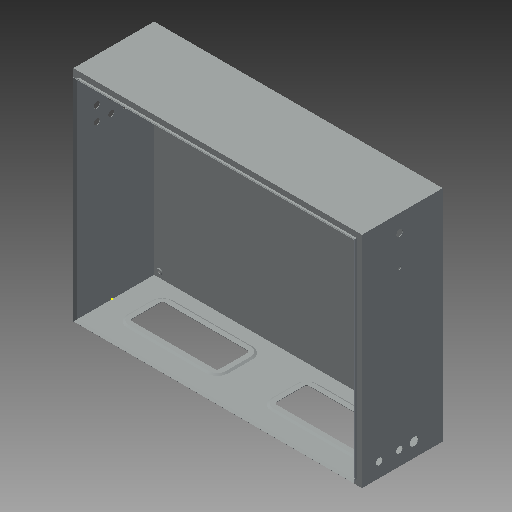
# Autodesk Inventor part: 1130_01_00 (2)
Saved by Autodesk Inventor 2019.3 (Build 233278000, 278)
## iProperties
Category: PARTsolutions
Company: RITTAL
Created: 2018-11-14
Part Number: 1130_01_00 (2)
Material: Generic
Catalog Web Link: www.cadenas.de
Description: Gehäusekorpus AE-Gehäusekorpus AE
Vendor: RITTAL
Document SubType Name: Modeling
Designer: psadmin
Manufacturer: RITTAL
Mass: 2682.24 g
Surface Area: 35840.6 cm^2
Volume: 2682.24 cm^3
Density: 1 g/cm^3
Appearance: PSOLRGB-195-201-196
PSOL_IDENT_0: {$CADENAS_DATA\23d-libs\rittal_usa\schaltschranksys\kompakt_schaltschr\ae\parts_ae\gehaeusekorpus_ae
PSOL_IDENT_1: .prj},204 {VTYP=3D},{NB=1130_01_00 (2)},{LINA=1130_01_00 (2)},{NN=Gehäusekorpus AE},{DATE=08.11.2018
PSOL_IDENT_2: 06:46:30},{GEOMDATE=18.08.2014 07:27:00},{VERSION=v140818072938},{LINEID=220},{WBVAR=DETAIL},{WBNUM
PSOL_IDENT_3: ERIC=DETAIL}  {NB=1130_01_00 (2)},{LINA=1130_01_00 (2)},{KT=DUMMY},{BEST=1130},{VER1=1},{VER2=1},{BE
PSOL_IDENT_4: Z1=MIN},{BEZ2=MIN},{BEZ3=MIN},{VER=1},{SS=1.50},{DETAIL=2},{A=1000.000},{B=760.000},{C=300.000},{D=3
PSOL_IDENT_5: 03.000},{E=113.000},{F=70.000},{G=30.000},{H=705.000},{I=667.200},{K=730.000},{P=905.000},{Q=944.000
PSOL_IDENT_6: },{R=495.000},{S=755.000},{T=616.400},{U=675.000},{V=27.000},{W=698.000},{X=0.000},{Y=0.000},{B1=100
PSOL_IDENT_7: 0},{H1=760},{T1=300},{F1=944},{G1=730},{S1=3.0},{GEW=56.0},{VERS=2},{GG=10.000},{AA=17.000},{BB=7.00
PSOL_IDENT_8: 0},{CC=10.000},{RR=31.000}
NN: Gehäusekorpus AE
NT: Gehäusekorpus AE
NB: 1130_01_00 (2)
NBSYN: $BEST._01_00 ($DETAIL.)
LINA: 1130_01_00 (2)
BEST: 1130
VER1: 1
VER2: 1
BEZ1: 0
BEZ2: 0
BEZ3: 0
VER: 1
SS: 1.5
DETAIL: 2
A: 1000
B: 760
C: 300
D: 303
E: 113
F: 70
G: 30
H: 705
I: 667.2
K: 730
P: 905
Q: 944
R: 495
S: 755
T: 616.4
U: 675
V: 27
W: 698
X: 0
Y: 0
B1: 1000
H1: 760
T1: 300
F1: 944
G1: 730
S1: 3
GEW: 56
VERS: 2
GG: 10
AA: 17
BB: 7
CC: 10
RR: 31
SUPPLIER: RITTAL
ARTICLENO: 1130_01_00 (2)
BOMINFO: 1130_01_00 (2)
CREATOR: CADENAS GmbH
Title: 1130_01_00 (2)
Author: Cadenas PARTsolutions
Comments: Gehäusekorpus AE
Autodesk Inventor part; units mm, degrees
sketch "Sketch_10" plane through (0, 0, 0) normal (0, 1, 0) x (-1, 0, 0)
  line L0 (500, 130) -> (-500, 130)
  line L1 (-500, 130) -> (-500, -150)
  line L2 (-500, -150) -> (500, -150)
  line L3 (500, -150) -> (500, 130)
  constraints: 8 end point
extrude "Extrusion1" add sketch "Sketch_10" along normal blind 760
sketch "Skizze_4" plane through (0, 0, 0) normal (1, 0, 0) x (0, 0, -1)
  line L0 (-300, 741) -> (-300, 19)
  line L1 (-300, 19) -> (0, 19)
  line L2 (0, 19) -> (0, 741)
  line L3 (0, 741) -> (-300, 741)
  constraints: 8 end point
extrude "Extrusion2" cut sketch "Skizze_4" along normal mid plane 961
sketch "Sketch_9" plane through (0, 0, 0) normal (1, 0, 0) x (0, 1, 0)
  line L0 (758.5, 128.5) -> (1.5, 128.5)
  line L1 (1.5, 128.5) -> (1.5, -148.5)
  line L2 (1.5, -148.5) -> (758.5, -148.5)
  line L3 (758.5, -148.5) -> (758.5, 128.5)
  constraints: 8 end point
extrude "Extrusion3" cut sketch "Sketch_9" along normal mid plane 997
sketch "Skizze_6" plane through (0, 0, 0) normal (1, 0, 0) x (0, 0, -1)
  line L0 (-144.3113, 14.6427) -> (-143.4081, 13.4441)
  line L1 (-143.4081, 13.4441) -> (-136.225, 18.5)
  line L2 (-136.225, 18.5) -> (-128.5, 18.5)
  line L3 (-128.5, 18.5) -> (-128.5, 20)
  line L4 (-128.5, 20) -> (-136.7, 20)
  line L5 (-136.7, 20) -> (-144.3113, 14.6427)
  constraints: 12 end point
extrude "Extrusion4" add sketch "Skizze_6" along normal mid plane 974.4
sketch "Skizze_7" plane through (0, 0, 0) normal (1, 0, 0) x (0, 0, -1)
  line L0 (-144.3113, 745.3573) -> (-136.7, 740)
  line L1 (-136.7, 740) -> (-128.5, 740)
  line L2 (-128.5, 740) -> (-128.5, 741.5)
  line L3 (-128.5, 741.5) -> (-136.225, 741.5)
  line L4 (-136.225, 741.5) -> (-143.4081, 746.5559)
  line L5 (-143.4081, 746.5559) -> (-144.3113, 745.3573)
  constraints: 12 end point
extrude "Extrusion5" add sketch "Skizze_7" along normal mid plane 973
sketch "Skizze_8" plane through (0, 380, 0) normal (0, 1, 0) x (1, 0, 0)
  line L0 (480, -136.7) -> (485.3573, -144.3113)
  line L1 (485.3573, -144.3113) -> (487.5552, -144.3113)
  line L2 (487.5552, -144.3113) -> (487.5552, -128.5)
  line L3 (487.5552, -128.5) -> (480, -128.5)
  line L4 (480, -128.5) -> (480, -136.7)
  constraints: 10 end point
extrude "Extrusion6" add sketch "Skizze_8" along normal mid plane 737.4
sketch "Skizze_9" plane through (0, 380, 0) normal (0, 1, 0) x (1, 0, 0)
  line L0 (-487.5552, -144.3113) -> (-485.3573, -144.3113)
  line L1 (-485.3573, -144.3113) -> (-480, -136.7)
  line L2 (-480, -136.7) -> (-480, -128.5)
  line L3 (-480, -128.5) -> (-487.5552, -128.5)
  line L4 (-487.5552, -128.5) -> (-487.5552, -144.3113)
  constraints: 10 end point
extrude "Extrusion7" add sketch "Skizze_9" along normal mid plane 737.4
sketch "Skizze_20" plane through (0, 0, 0) normal (1, 0, 0) x (0, 0, -1)
  line L0 (-439.6277, 761.5) -> (-439.6277, -1.5)
  line L1 (-439.6277, -1.5) -> (-130, -1.5)
  line L2 (-130, -1.5) -> (-130, 18.5)
  line L3 (-130, 18.5) -> (-136.225, 18.5)
  line L4 (-136.225, 18.5) -> (-143.4081, 13.4441)
  line L5 (-143.4081, 13.4441) -> (-419.6277, 380)
  line L6 (-419.6277, 380) -> (-143.4081, 746.5559)
  line L7 (-143.4081, 746.5559) -> (-136.225, 741.5)
  line L8 (-136.225, 741.5) -> (-130, 741.5)
  line L9 (-130, 741.5) -> (-130, 761.5)
  line L10 (-130, 761.5) -> (-439.6277, 761.5)
  constraints: 22 end point
extrude "Extrusion8" cut sketch "Skizze_20" along normal mid plane 1973
sketch "Skizze_21" plane through (0, 380, 0) normal (0, 1, 0) x (1, 0, 0)
  line L0 (-501.5, -530.0542) -> (501.5, -530.0542)
  line L1 (501.5, -530.0542) -> (501.5, -130)
  line L2 (501.5, -130) -> (481.5, -130)
  line L3 (481.5, -130) -> (481.5, -136.225)
  line L4 (481.5, -136.225) -> (486.5559, -143.4081)
  line L5 (486.5559, -143.4081) -> (0, -510.0542)
  line L6 (0, -510.0542) -> (-486.5559, -143.4081)
  line L7 (-486.5559, -143.4081) -> (-481.5, -136.225)
  line L8 (-481.5, -136.225) -> (-481.5, -130)
  line L9 (-481.5, -130) -> (-501.5, -130)
  line L10 (-501.5, -130) -> (-501.5, -530.0542)
  constraints: 22 end point
extrude "Extrusion9" cut sketch "Skizze_21" along normal mid plane 752.4
sketch "Skizze_28" plane through (0, 0, 0) normal (0, 1, 0) x (1, 0, 0)
  arc A0 (-432.9449, -16.4449) -> (-384.9449, -64.4449) centre (-384.9449, -16.4449) ccw
  line L0 (-384.9449, -64.4449) -> (-115.0551, -64.4449)
  arc A1 (-115.0551, -64.4449) -> (-67.0551, -16.4449) centre (-115.0551, -16.4449) ccw
  line L1 (-67.0551, -16.4449) -> (-67.0551, 63.4449)
  arc A2 (-67.0551, 63.4449) -> (-115.0551, 111.4449) centre (-115.0551, 63.4449) ccw
  line L2 (-115.0551, 111.4449) -> (-384.9449, 111.4449)
  arc A3 (-384.9449, 111.4449) -> (-432.9449, 63.4449) centre (-384.9449, 63.4449) ccw
  line L3 (-432.9449, 63.4449) -> (-432.9449, -16.4449)
  constraints: 8 end point, 8 point on circle, 4 centre point
extrude "Extrusion10" cut sketch "Skizze_28" along normal blind 1.5
sketch "Skizze_29" plane through (0, 0, -23.5) normal (0, 0, 1) x (1, 0, 0)
  line L0 (-102.5, 5.5) -> (-102.5, 4)
  line L1 (-102.5, 4) -> (-81.9019, 4)
  line L2 (-81.9019, 4) -> (-74.9737, 0)
  line L3 (-74.9737, 0) -> (-66.7551, 0)
  line L4 (-66.7551, 0) -> (-66.7551, 1.5)
  line L5 (-66.7551, 1.5) -> (-74.5718, 1.5)
  line L6 (-74.5718, 1.5) -> (-81.5, 5.5)
  line L7 (-81.5, 5.5) -> (-102.5, 5.5)
  constraints: 16 end point
extrude "Extrusion11" add sketch "Skizze_29" along normal mid plane 85
sketch "Skizze_30" plane through (0, 0, -23.5) normal (0, 0, 1) x (1, 0, 0)
  line L0 (-433.2449, 1.5) -> (-433.2449, 0)
  line L1 (-433.2449, 0) -> (-425.3263, 0)
  line L2 (-425.3263, 0) -> (-418.3981, 4)
  line L3 (-418.3981, 4) -> (-397.8, 4)
  line L4 (-397.8, 4) -> (-397.8, 5.5)
  line L5 (-397.8, 5.5) -> (-418.8, 5.5)
  line L6 (-418.8, 5.5) -> (-425.7282, 1.5)
  line L7 (-425.7282, 1.5) -> (-433.2449, 1.5)
  constraints: 16 end point
extrude "Extrusion12" add sketch "Skizze_30" along normal mid plane 85
sketch "Skizze_31" plane through (0, 0, -66) normal (0, 0, 1) x (1, 0, 0)
  line L0 (-112.5, -50) -> (-112.5, 50)
  line L1 (-102.5, 5.5) -> (-102.5, 4)
  line L2 (-102.5, 4) -> (-81.9019, 4)
  line L3 (-81.9019, 4) -> (-74.9737, 0)
  line L4 (-74.9737, 0) -> (-66.7551, 0)
  line L5 (-66.7551, 0) -> (-66.7551, 1.5)
  line L6 (-66.7551, 1.5) -> (-74.5718, 1.5)
  line L7 (-74.5718, 1.5) -> (-81.5, 5.5)
  line L8 (-81.5, 5.5) -> (-102.5, 5.5)
  constraints: 18 end point
revolve "Revolution1" add sketch "Skizze_31" angle 90 about axis through (-112.5, -50, -66) along (0, 1, 0)
sketch "Skizze_32" plane through (0, 0, -66) normal (0, 0, 1) x (1, 0, 0)
  line L0 (-387.5, 4) -> (-387.5, -4)
  line L1 (-433.2449, 1.5) -> (-433.2449, 0)
  line L2 (-433.2449, 0) -> (-425.0263, 0)
  line L3 (-425.0263, 0) -> (-418.0981, 4)
  line L4 (-418.0981, 4) -> (-397.5, 4)
  line L5 (-397.5, 4) -> (-397.5, 5.5)
  line L6 (-397.5, 5.5) -> (-418.5, 5.5)
  line L7 (-418.5, 5.5) -> (-425.4282, 1.5)
  line L8 (-425.4282, 1.5) -> (-433.2449, 1.5)
  constraints: 18 end point
revolve "Revolution2" add sketch "Skizze_32" angle 90 about axis through (-387.5, 4, -66) along (0, -1, 0)
sketch "Skizze_33" plane through (0, 0, 19) normal (0, 0, 1) x (1, 0, 0)
  line L0 (-112.5, -50) -> (-112.5, 50)
  line L1 (-102.5, 5.5) -> (-102.5, 4)
  line L2 (-102.5, 4) -> (-81.9019, 4)
  line L3 (-81.9019, 4) -> (-74.9737, 0)
  line L4 (-74.9737, 0) -> (-66.7551, 0)
  line L5 (-66.7551, 0) -> (-66.7551, 1.5)
  line L6 (-66.7551, 1.5) -> (-74.5718, 1.5)
  line L7 (-74.5718, 1.5) -> (-81.5, 5.5)
  line L8 (-81.5, 5.5) -> (-102.5, 5.5)
  constraints: 18 end point
revolve "Revolution3" add sketch "Skizze_33" angle 90 about axis through (-112.5, -50, 19) along (0, -1, 0)
sketch "Skizze_34" plane through (0, 0, 19) normal (0, 0, 1) x (1, 0, 0)
  line L0 (-387.5, 4) -> (-387.5, -4)
  line L1 (-433.2449, 1.5) -> (-433.2449, 0)
  line L2 (-433.2449, 0) -> (-425.0263, 0)
  line L3 (-425.0263, 0) -> (-418.0981, 4)
  line L4 (-418.0981, 4) -> (-397.5, 4)
  line L5 (-397.5, 4) -> (-397.5, 5.5)
  line L6 (-397.5, 5.5) -> (-418.5, 5.5)
  line L7 (-418.5, 5.5) -> (-425.4282, 1.5)
  line L8 (-425.4282, 1.5) -> (-433.2449, 1.5)
  constraints: 18 end point
revolve "Revolution4" add sketch "Skizze_34" angle 90 about axis through (-387.5, 4, 19) along (0, 1, 0)
sketch "Skizze_35" plane through (-250, 0, 0) normal (1, 0, 0) x (0, 0, -1)
  line L0 (76, 5.5) -> (76, 4)
  line L1 (76, 4) -> (96.5981, 4)
  line L2 (96.5981, 4) -> (103.5263, 0)
  line L3 (103.5263, 0) -> (111.7449, 0)
  line L4 (111.7449, 0) -> (111.7449, 1.5)
  line L5 (111.7449, 1.5) -> (103.9282, 1.5)
  line L6 (103.9282, 1.5) -> (97, 5.5)
  line L7 (97, 5.5) -> (76, 5.5)
  constraints: 16 end point
extrude "Extrusion13" add sketch "Skizze_35" along normal mid plane 275
sketch "Skizze_36" plane through (-250, 0, 0) normal (1, 0, 0) x (0, 0, -1)
  line L0 (-64.7449, 1.5) -> (-64.7449, 0)
  line L1 (-64.7449, 0) -> (-56.5263, 0)
  line L2 (-56.5263, 0) -> (-49.5981, 4)
  line L3 (-49.5981, 4) -> (-29, 4)
  line L4 (-29, 4) -> (-29, 5.5)
  line L5 (-29, 5.5) -> (-50, 5.5)
  line L6 (-50, 5.5) -> (-56.9282, 1.5)
  line L7 (-56.9282, 1.5) -> (-64.7449, 1.5)
  constraints: 16 end point
extrude "Extrusion14" add sketch "Skizze_36" along normal mid plane 275
sketch "Skizze_105" plane through (0, 5.5, 0) normal (0, 1, 0) x (1, 0, 0)
  line L0 (-401.5, -33) -> (-98.5, -33)
  line L1 (-98.5, -33) -> (-98.5, 80)
  line L2 (-98.5, 80) -> (-401.5, 80)
  line L3 (-401.5, 80) -> (-401.5, -33)
  constraints: 8 end point
extrude "Extrusion15" add sketch "Skizze_105" against normal blind 1.5
sketch "Skizze_106" plane through (0, 5.5, 0) normal (0, 1, 0) x (1, 0, 0)
  arc A0 (-401.5, -25) -> (-393.5, -33) centre (-393.5, -25) ccw
  line L0 (-393.5, -33) -> (-106.5, -33)
  arc A1 (-106.5, -33) -> (-98.5, -25) centre (-106.5, -25) ccw
  line L1 (-98.5, -25) -> (-98.5, 72)
  arc A2 (-98.5, 72) -> (-106.5, 80) centre (-106.5, 72) ccw
  line L2 (-106.5, 80) -> (-393.5, 80)
  arc A3 (-393.5, 80) -> (-401.5, 72) centre (-393.5, 72) ccw
  line L3 (-401.5, 72) -> (-401.5, -25)
  constraints: 8 end point, 8 point on circle, 4 centre point
extrude "Extrusion16" cut sketch "Skizze_106" against normal blind 1.5
sketch "Skizze_37" plane through (0, 0, 0) normal (0, 1, 0) x (1, 0, 0)
  arc A0 (67.0551, -16.4449) -> (115.0551, -64.4449) centre (115.0551, -16.4449) ccw
  line L0 (115.0551, -64.4449) -> (384.9449, -64.4449)
  arc A1 (384.9449, -64.4449) -> (432.9449, -16.4449) centre (384.9449, -16.4449) ccw
  line L1 (432.9449, -16.4449) -> (432.9449, 63.4449)
  arc A2 (432.9449, 63.4449) -> (384.9449, 111.4449) centre (384.9449, 63.4449) ccw
  line L2 (384.9449, 111.4449) -> (115.0551, 111.4449)
  arc A3 (115.0551, 111.4449) -> (67.0551, 63.4449) centre (115.0551, 63.4449) ccw
  line L3 (67.0551, 63.4449) -> (67.0551, -16.4449)
  constraints: 8 end point, 8 point on circle, 4 centre point
extrude "Extrusion17" cut sketch "Skizze_37" along normal blind 1.5
sketch "Skizze_38" plane through (0, 0, -23.5) normal (0, 0, 1) x (1, 0, 0)
  line L0 (397.5, 5.5) -> (397.5, 4)
  line L1 (397.5, 4) -> (418.0981, 4)
  line L2 (418.0981, 4) -> (425.0263, 0)
  line L3 (425.0263, 0) -> (433.2449, 0)
  line L4 (433.2449, 0) -> (433.2449, 1.5)
  line L5 (433.2449, 1.5) -> (425.4282, 1.5)
  line L6 (425.4282, 1.5) -> (418.5, 5.5)
  line L7 (418.5, 5.5) -> (397.5, 5.5)
  constraints: 16 end point
extrude "Extrusion18" add sketch "Skizze_38" along normal mid plane 85
sketch "Skizze_39" plane through (0, 0, -23.5) normal (0, 0, 1) x (1, 0, 0)
  line L0 (66.7551, 1.5) -> (66.7551, 0)
  line L1 (66.7551, 0) -> (74.9737, 0)
  line L2 (74.9737, 0) -> (81.9019, 4)
  line L3 (81.9019, 4) -> (102.5, 4)
  line L4 (102.5, 4) -> (102.5, 5.5)
  line L5 (102.5, 5.5) -> (81.5, 5.5)
  line L6 (81.5, 5.5) -> (74.5718, 1.5)
  line L7 (74.5718, 1.5) -> (66.7551, 1.5)
  constraints: 16 end point
extrude "Extrusion19" add sketch "Skizze_39" along normal mid plane 85
sketch "Skizze_40" plane through (0, 0, -66) normal (0, 0, 1) x (1, 0, 0)
  line L0 (387.5, -4) -> (387.5, 4)
  line L1 (397.5, 5.5) -> (397.5, 4)
  line L2 (397.5, 4) -> (418.0981, 4)
  line L3 (418.0981, 4) -> (425.0263, 0)
  line L4 (425.0263, 0) -> (433.2449, 0)
  line L5 (433.2449, 0) -> (433.2449, 1.5)
  line L6 (433.2449, 1.5) -> (425.4282, 1.5)
  line L7 (425.4282, 1.5) -> (418.5, 5.5)
  line L8 (418.5, 5.5) -> (397.5, 5.5)
  constraints: 18 end point
revolve "Revolution5" add sketch "Skizze_40" angle 90 about axis through (387.5, -4, -66) along (0, 1, 0)
sketch "Skizze_41" plane through (0, 0, -66) normal (0, 0, 1) x (1, 0, 0)
  line L0 (112.5, 4) -> (112.5, -4)
  line L1 (66.7551, 1.5) -> (66.7551, 0)
  line L2 (66.7551, 0) -> (74.9737, 0)
  line L3 (74.9737, 0) -> (81.9019, 4)
  line L4 (81.9019, 4) -> (102.5, 4)
  line L5 (102.5, 4) -> (102.5, 5.5)
  line L6 (102.5, 5.5) -> (81.5, 5.5)
  line L7 (81.5, 5.5) -> (74.5718, 1.5)
  line L8 (74.5718, 1.5) -> (66.7551, 1.5)
  constraints: 18 end point
revolve "Revolution6" add sketch "Skizze_41" angle 90 about axis through (112.5, 4, -66) along (0, -1, 0)
sketch "Skizze_42" plane through (0, 0, 19) normal (0, 0, 1) x (1, 0, 0)
  line L0 (387.5, -4) -> (387.5, 4)
  line L1 (397.5, 5.5) -> (397.5, 4)
  line L2 (397.5, 4) -> (418.0981, 4)
  line L3 (418.0981, 4) -> (425.0263, 0)
  line L4 (425.0263, 0) -> (433.2449, 0)
  line L5 (433.2449, 0) -> (433.2449, 1.5)
  line L6 (433.2449, 1.5) -> (425.4282, 1.5)
  line L7 (425.4282, 1.5) -> (418.5, 5.5)
  line L8 (418.5, 5.5) -> (397.5, 5.5)
  constraints: 18 end point
revolve "Revolution7" add sketch "Skizze_42" angle 90 about axis through (387.5, -4, 19) along (0, -1, 0)
sketch "Skizze_43" plane through (0, 0, 19) normal (0, 0, 1) x (1, 0, 0)
  line L0 (112.5, 4) -> (112.5, -4)
  line L1 (66.7551, 1.5) -> (66.7551, 0)
  line L2 (66.7551, 0) -> (74.9737, 0)
  line L3 (74.9737, 0) -> (81.9019, 4)
  line L4 (81.9019, 4) -> (102.5, 4)
  line L5 (102.5, 4) -> (102.5, 5.5)
  line L6 (102.5, 5.5) -> (81.5, 5.5)
  line L7 (81.5, 5.5) -> (74.5718, 1.5)
  line L8 (74.5718, 1.5) -> (66.7551, 1.5)
  constraints: 18 end point
revolve "Revolution8" add sketch "Skizze_43" angle 90 about axis through (112.5, 4, 19) along (0, 1, 0)
sketch "Skizze_44" plane through (250, 0, 0) normal (1, 0, 0) x (0, 0, -1)
  line L0 (76, 5.5) -> (76, 4)
  line L1 (76, 4) -> (96.5981, 4)
  line L2 (96.5981, 4) -> (103.5263, 0)
  line L3 (103.5263, 0) -> (111.7449, 0)
  line L4 (111.7449, 0) -> (111.7449, 1.5)
  line L5 (111.7449, 1.5) -> (103.9282, 1.5)
  line L6 (103.9282, 1.5) -> (97, 5.5)
  line L7 (97, 5.5) -> (76, 5.5)
  constraints: 16 end point
extrude "Extrusion20" add sketch "Skizze_44" along normal mid plane 275
sketch "Skizze_45" plane through (250, 0, 0) normal (1, 0, 0) x (0, 0, -1)
  line L0 (-64.7449, 1.5) -> (-64.7449, 0)
  line L1 (-64.7449, 0) -> (-56.5263, 0)
  line L2 (-56.5263, 0) -> (-49.5981, 4)
  line L3 (-49.5981, 4) -> (-29, 4)
  line L4 (-29, 4) -> (-29, 5.5)
  line L5 (-29, 5.5) -> (-50, 5.5)
  line L6 (-50, 5.5) -> (-56.9282, 1.5)
  line L7 (-56.9282, 1.5) -> (-64.7449, 1.5)
  constraints: 16 end point
extrude "Extrusion21" add sketch "Skizze_45" along normal mid plane 275
sketch "Skizze_107" plane through (0, 5.5, 0) normal (0, 1, 0) x (1, 0, 0)
  line L0 (98.5, -33) -> (401.5, -33)
  line L1 (401.5, -33) -> (401.5, 80)
  line L2 (401.5, 80) -> (98.5, 80)
  line L3 (98.5, 80) -> (98.5, -33)
  constraints: 8 end point
extrude "Extrusion22" add sketch "Skizze_107" against normal blind 1.5
sketch "Skizze_108" plane through (0, 5.5, 0) normal (0, 1, 0) x (1, 0, 0)
  arc A0 (98.5, -25) -> (106.5, -33) centre (106.5, -25) ccw
  line L0 (106.5, -33) -> (393.5, -33)
  arc A1 (393.5, -33) -> (401.5, -25) centre (393.5, -25) ccw
  line L1 (401.5, -25) -> (401.5, 72)
  arc A2 (401.5, 72) -> (393.5, 80) centre (393.5, 72) ccw
  line L2 (393.5, 80) -> (106.5, 80)
  arc A3 (106.5, 80) -> (98.5, 72) centre (106.5, 72) ccw
  line L3 (98.5, 72) -> (98.5, -25)
  constraints: 8 end point, 8 point on circle, 4 centre point
extrude "Extrusion23" cut sketch "Skizze_108" against normal blind 1.5
sketch "Sketch32" plane through (500, 0, -150) normal (0, 0, -1) x (-1, 0, 0)
  point P0 (20, 20)
hole "Hole1" at (480, 20, -150) direction (0, 0, 1) diameter 24 depth 1.5
sketch "Sketch33" plane through (500, 0, -150) normal (0, 0, -1) x (-1, 0, 0)
  point P0 (20, 740)
hole "Hole2" at (480, 740, -150) direction (0, 0, 1) diameter 24 depth 1.5
sketch "Skizze_68" plane through (480, 0, 0) normal (1, 0, 0) x (0, 0, -1)
  line L0 (150, 20) -> (148.5, 20)
  line L1 (146.5, 28.6213) -> (146.5, 24.35)
  line L2 (146.5, 24.35) -> (148, 24.35)
  line L3 (148, 24.35) -> (148, 28)
  line L4 (148, 28) -> (150, 30)
  line L5 (150, 30) -> (150, 32.5)
  line L6 (150, 32.5) -> (148.5, 32.5)
  line L7 (148.5, 32.5) -> (148.5, 30.6213)
  line L8 (148.5, 30.6213) -> (146.5, 28.6213)
  constraints: 18 end point
revolve "Revolution9" add sketch "Skizze_68" angle 360 about axis through (480, 20, -150) along (0, 0, -1)
sketch "Skizze_71" plane through (480, 0, 0) normal (1, 0, 0) x (0, 0, -1)
  line L0 (150, 740) -> (148.5, 740)
  line L1 (146.5, 748.6213) -> (146.5, 744.35)
  line L2 (146.5, 744.35) -> (148, 744.35)
  line L3 (148, 744.35) -> (148, 748)
  line L4 (148, 748) -> (150, 750)
  line L5 (150, 750) -> (150, 752.5)
  line L6 (150, 752.5) -> (148.5, 752.5)
  line L7 (148.5, 752.5) -> (148.5, 750.6213)
  line L8 (148.5, 750.6213) -> (146.5, 748.6213)
  constraints: 18 end point
revolve "Revolution10" add sketch "Skizze_71" angle 360 about axis through (480, 740, -150) along (0, 0, -1)
sketch "Sketch36" plane through (500, 0, -150) normal (0, 0, -1) x (-1, 0, 0)
  point P0 (980, 20)
hole "Hole3" at (-480, 20, -150) direction (0, 0, 1) diameter 24 depth 1.5
sketch "Sketch37" plane through (500, 0, -150) normal (0, 0, -1) x (-1, 0, 0)
  point P0 (980, 740)
hole "Hole4" at (-480, 740, -150) direction (0, 0, 1) diameter 24 depth 1.5
sketch "Skizze_75" plane through (-480, 0, 0) normal (1, 0, 0) x (0, 0, -1)
  line L0 (150, 20) -> (148.5, 20)
  line L1 (146.5, 28.6213) -> (146.5, 24.35)
  line L2 (146.5, 24.35) -> (148, 24.35)
  line L3 (148, 24.35) -> (148, 28)
  line L4 (148, 28) -> (150, 30)
  line L5 (150, 30) -> (150, 32.5)
  line L6 (150, 32.5) -> (148.5, 32.5)
  line L7 (148.5, 32.5) -> (148.5, 30.6213)
  line L8 (148.5, 30.6213) -> (146.5, 28.6213)
  constraints: 18 end point
revolve "Revolution11" add sketch "Skizze_75" angle 360 about axis through (-480, 20, -150) along (0, 0, -1)
sketch "Skizze_76" plane through (-480, 0, 0) normal (1, 0, 0) x (0, 0, -1)
  line L0 (150, 740) -> (148.5, 740)
  line L1 (146.5, 748.6213) -> (146.5, 744.35)
  line L2 (146.5, 744.35) -> (148, 744.35)
  line L3 (148, 744.35) -> (148, 748)
  line L4 (148, 748) -> (150, 750)
  line L5 (150, 750) -> (150, 752.5)
  line L6 (150, 752.5) -> (148.5, 752.5)
  line L7 (148.5, 752.5) -> (148.5, 750.6213)
  line L8 (148.5, 750.6213) -> (146.5, 748.6213)
  constraints: 18 end point
revolve "Revolution12" add sketch "Skizze_76" angle 360 about axis through (-480, 740, -150) along (0, 0, -1)
ref_plane "DPB11_XY" through (500, 380, 0) normal (0, 0, 1) x (1, 0, 0)
ref_plane "DPB11_YZ" through (500, 380, 0) normal (1, 0, 0) x (0, 1, 0)
ref_plane "DPB11_ZX" through (500, 380, 0) normal (0, 1, 0) x (0, 0, 1)
ref_plane "DPB12_XY" through (-500, 380, 0) normal (0, 0, 1) x (1, 0, 0)
ref_plane "DPB12_YZ" through (-500, 380, 0) normal (1, 0, 0) x (0, 1, 0)
ref_plane "DPB12_ZX" through (-500, 380, 0) normal (0, 1, 0) x (0, 0, 1)
ref_plane "DPB61_XY" through (-401.5, 4, 0) normal (0, 0, 1) x (1, 0, 0)
ref_plane "DPB61_YZ" through (-401.5, 4, 0) normal (1, 0, 0) x (0, 1, 0)
ref_plane "DPB61_ZX" through (-401.5, 4, 0) normal (0, 1, 0) x (0, 0, 1)
ref_plane "DPB611_XY" through (98.5, 4, 0) normal (0, 0, 1) x (1, 0, 0)
ref_plane "DPB611_YZ" through (98.5, 4, 0) normal (1, 0, 0) x (0, 1, 0)
ref_plane "DPB611_ZX" through (98.5, 4, 0) normal (0, 1, 0) x (0, 0, 1)
ref_plane "DPB62_XY" through (-98.5, 4, 0) normal (0, 0, 1) x (1, 0, 0)
ref_plane "DPB62_YZ" through (-98.5, 4, 0) normal (1, 0, 0) x (0, 1, 0)
ref_plane "DPB62_ZX" through (-98.5, 4, 0) normal (0, 1, 0) x (0, 0, 1)
ref_plane "DPB622_XY" through (401.5, 4, 0) normal (0, 0, 1) x (1, 0, 0)
ref_plane "DPB622_YZ" through (401.5, 4, 0) normal (1, 0, 0) x (0, 1, 0)
ref_plane "DPB622_ZX" through (401.5, 4, 0) normal (0, 1, 0) x (0, 0, 1)
ref_plane "DPH11_XY" through (0, 0, 0) normal (0, 0, 1) x (1, 0, 0)
ref_plane "DPH11_YZ" through (0, 0, 0) normal (1, 0, 0) x (0, 1, 0)
ref_plane "DPH11_ZX" through (0, 0, 0) normal (0, 1, 0) x (0, 0, 1)
ref_plane "DPH12_XY" through (0, 760, 0) normal (0, 0, 1) x (1, 0, 0)
ref_plane "DPH12_YZ" through (0, 760, 0) normal (1, 0, 0) x (0, 1, 0)
ref_plane "DPH12_ZX" through (0, 760, 0) normal (0, 1, 0) x (0, 0, 1)
ref_plane "DPH21_XY" through (0, 2.5, 150) normal (1, 0, 0) x (0, 0, -1)
ref_plane "DPH21_YZ" through (0, 2.5, 150) normal (0, 0, -1) x (0, 1, 0)
ref_plane "DPH21_ZX" through (0, 2.5, 150) normal (0, 1, 0) x (1, 0, 0)
ref_plane "DPH22_XY" through (0, 757.5, 150) normal (1, 0, 0) x (0, 0, -1)
ref_plane "DPH22_YZ" through (0, 757.5, 150) normal (0, 0, -1) x (0, 1, 0)
ref_plane "DPH22_ZX" through (0, 757.5, 150) normal (0, 1, 0) x (1, 0, 0)
ref_plane "DPH31_XY" through (0, 20, 136.5) normal (1, 0, 0) x (0, 0, -1)
ref_plane "DPH31_YZ" through (0, 20, 136.5) normal (0, 0, -1) x (0, 1, 0)
ref_plane "DPH31_ZX" through (0, 20, 136.5) normal (0, 1, 0) x (1, 0, 0)
ref_plane "DPH32_XY" through (0, 740, 136.5) normal (1, 0, 0) x (0, 0, -1)
ref_plane "DPH32_YZ" through (0, 740, 136.5) normal (0, 0, -1) x (0, 1, 0)
ref_plane "DPH32_ZX" through (0, 740, 136.5) normal (0, 1, 0) x (1, 0, 0)
ref_plane "DPH51_XY" through (0, 0, -150) normal (1, 0, 0) x (0, 0, -1)
ref_plane "DPH51_YZ" through (0, 0, -150) normal (0, 0, -1) x (0, 1, 0)
ref_plane "DPH51_ZX" through (0, 0, -150) normal (0, 1, 0) x (1, 0, 0)
ref_plane "DPH52_XY" through (0, 30, -150) normal (1, 0, 0) x (0, 0, -1)
ref_plane "DPH52_YZ" through (0, 30, -150) normal (0, 0, -1) x (0, 1, 0)
ref_plane "DPH52_ZX" through (0, 30, -150) normal (0, 1, 0) x (1, 0, 0)
ref_plane "DPH61_XY" through (0, 2.5, 150) normal (1, 0, 0) x (0, 0, -1)
ref_plane "DPH61_YZ" through (0, 2.5, 150) normal (0, 0, -1) x (0, 1, 0)
ref_plane "DPH61_ZX" through (0, 2.5, 150) normal (0, 1, 0) x (1, 0, 0)
ref_plane "DPH62_XY" through (0, 0, 130) normal (1, 0, 0) x (0, 0, -1)
ref_plane "DPH62_YZ" through (0, 0, 130) normal (0, 0, -1) x (0, 1, 0)
ref_plane "DPH62_ZX" through (0, 0, 130) normal (0, 1, 0) x (1, 0, 0)
ref_plane "DPT11_XY" through (0, 0, -150) normal (1, 0, 0) x (0, 0, -1)
ref_plane "DPT11_YZ" through (0, 0, -150) normal (0, 0, -1) x (0, 1, 0)
ref_plane "DPT11_ZX" through (0, 0, -150) normal (0, 1, 0) x (1, 0, 0)
ref_plane "DPT12_XY" through (0, 2.5, 150) normal (1, 0, 0) x (0, 0, -1)
ref_plane "DPT12_YZ" through (0, 2.5, 150) normal (0, 0, -1) x (0, 1, 0)
ref_plane "DPT12_ZX" through (0, 2.5, 150) normal (0, 1, 0) x (1, 0, 0)
ref_plane "DPT21_XY" through (0, 760, -150) normal (1, 0, 0) x (0, 0, -1)
ref_plane "DPT21_YZ" through (0, 760, -150) normal (0, 0, -1) x (0, 1, 0)
ref_plane "DPT21_ZX" through (0, 760, -150) normal (0, 1, 0) x (1, 0, 0)
ref_plane "DPT22_XY" through (0, 760, 130) normal (1, 0, 0) x (0, 0, -1)
ref_plane "DPT22_YZ" through (0, 760, 130) normal (0, 0, -1) x (0, 1, 0)
ref_plane "DPT22_ZX" through (0, 760, 130) normal (0, 1, 0) x (1, 0, 0)
ref_plane "DPT41_XY" through (0, 4, -150) normal (1, 0, 0) x (0, 0, -1)
ref_plane "DPT41_YZ" through (0, 4, -150) normal (0, 0, -1) x (0, 1, 0)
ref_plane "DPT41_ZX" through (0, 4, -150) normal (0, 1, 0) x (1, 0, 0)
ref_plane "DPT42_XY" through (0, 4, -80) normal (1, 0, 0) x (0, 0, -1)
ref_plane "DPT42_YZ" through (0, 4, -80) normal (0, 0, -1) x (0, 1, 0)
ref_plane "DPT42_ZX" through (0, 4, -80) normal (0, 1, 0) x (1, 0, 0)
ref_plane "DPT51_XY" through (0, 4, -80) normal (1, 0, 0) x (0, 0, -1)
ref_plane "DPT51_YZ" through (0, 4, -80) normal (0, 0, -1) x (0, 1, 0)
ref_plane "DPT51_ZX" through (0, 4, -80) normal (0, 1, 0) x (1, 0, 0)
ref_plane "DPT52_XY" through (0, 4, 33) normal (1, 0, 0) x (0, 0, -1)
ref_plane "DPT52_YZ" through (0, 4, 33) normal (0, 0, -1) x (0, 1, 0)
ref_plane "DPT52_ZX" through (0, 4, 33) normal (0, 1, 0) x (1, 0, 0)
ref_plane "flanschplatte_XY" through (-250, 0, -23.5) normal (0, 1, 0) x (1, 0, 0)
ref_plane "flanschplatte_YZ" through (-250, 0, -23.5) normal (1, 0, 0) x (0, 0, -1)
ref_plane "flanschplatte_ZX" through (-250, 0, -23.5) normal (0, 0, -1) x (0, 1, 0)
ref_plane "flanschplatte_2_XY" through (250, 0, -23.5) normal (0, 1, 0) x (1, 0, 0)
ref_plane "flanschplatte_2_YZ" through (250, 0, -23.5) normal (1, 0, 0) x (0, 0, -1)
ref_plane "flanschplatte_2_ZX" through (250, 0, -23.5) normal (0, 0, -1) x (0, 1, 0)
ref_plane "gehaeuse_XY" through (0, 0, 0) normal (0, 1, 0) x (1, 0, 0)
ref_plane "gehaeuse_YZ" through (0, 0, 0) normal (1, 0, 0) x (0, 0, -1)
ref_plane "gehaeuse_ZX" through (0, 0, 0) normal (0, 0, -1) x (0, 1, 0)
ref_plane "montageplatte_XY" through (-452.5, 30, -125.7) normal (0, 0, 1) x (1, 0, 0)
ref_plane "montageplatte_YZ" through (-452.5, 30, -125.7) normal (1, 0, 0) x (0, 1, 0)
ref_plane "montageplatte_ZX" through (-452.5, 30, -125.7) normal (0, 1, 0) x (0, 0, 1)
ref_plane "scharnier_o_XY" through (490.3, 691.85, 130) normal (0, 0, 1) x (1, 0, 0)
ref_plane "scharnier_o_YZ" through (490.3, 691.85, 130) normal (1, 0, 0) x (0, 1, 0)
ref_plane "scharnier_o_ZX" through (490.3, 691.85, 130) normal (0, 1, 0) x (0, 0, 1)
ref_plane "scharnier_o_links_XY" through (-490.3, 691.85, 130) normal (0, 0, 1) x (1, 0, 0)
ref_plane "scharnier_o_links_YZ" through (-490.3, 691.85, 130) normal (1, 0, 0) x (0, 1, 0)
ref_plane "scharnier_o_links_ZX" through (-490.3, 691.85, 130) normal (0, 1, 0) x (0, 0, 1)
ref_plane "scharnier_u_XY" through (490.3, 50.65, 130) normal (0, 0, 1) x (1, 0, 0)
ref_plane "scharnier_u_YZ" through (490.3, 50.65, 130) normal (1, 0, 0) x (0, 1, 0)
ref_plane "scharnier_u_ZX" through (490.3, 50.65, 130) normal (0, 1, 0) x (0, 0, 1)
ref_plane "scharnier_u_links_XY" through (-490.3, 50.65, 130) normal (0, 0, 1) x (1, 0, 0)
ref_plane "scharnier_u_links_YZ" through (-490.3, 50.65, 130) normal (1, 0, 0) x (0, 1, 0)
ref_plane "scharnier_u_links_ZX" through (-490.3, 50.65, 130) normal (0, 1, 0) x (0, 0, 1)
sketch "Эскиз40" plane through (-500, 0, -150) normal (-1, 0, 0) x (0, 0, 1)
  circle A0 centre (50, 610) radius 10.5
  line L0 (0, 760) -> (280, 760) projected
  line L1 (0, 0) -> (0, 760) projected
  point P0 (150, 0)
  dimension "d93" = 21
  dimension "d102" = 150
  dimension "d103" = 50
  constraints: 1 centre point
  measures "d93" diameter of A0
  measures "d102" distance from line of L0 A0.centre
  measures "d103" distance from line of L1 A0.centre
extrude "Выдавливание24" cut sketch "Эскиз40" against normal blind 10
pattern_linear "Прямоуг.массив1" count 4 spacing 50 along (0, 0, 1) count 2 spacing -50 along (0, 1, 0) of "Выдавливание24"
sketch "Эскиз41" plane through (-500, 0, -150) normal (-1, 0, 0) x (0, 0, 1)
  point P0 (150, 0)
sketch "Эскиз42" plane through (500, 0, 130) normal (1, 0, 0) x (0, 0, -1)
  circle A0 centre (130, 50) radius 11.5
  line L0 (280, 0) -> (280, 760) projected
  line L1 (0, 0) -> (280, 0) projected
  point P0 (130, 0)
  dimension "d104" = 23
  dimension "d105" = 150
  dimension "d106" = 50
  constraints: 1 centre point
  measures "d104" diameter of A0
  measures "d105" distance from line of L0 A0.centre
  measures "d106" distance from line of L1 A0.centre
extrude "Выдавливание25" cut sketch "Эскиз42" against normal blind 10
sketch "Эскиз43" plane through (500, 0, 130) normal (1, 0, 0) x (0, 0, -1)
  circle A0 centre (130, 595) radius 5
  line L0 (280, 0) -> (280, 760) projected
  line L1 (0, 760) -> (280, 760) projected
  point P0 (130, 0)
  dimension "d109" = 10
  dimension "d110" = 150
  dimension "d111" = 165
  constraints: 1 centre point
  measures "d109" diameter of A0
  measures "d110" distance from line of L0 A0.centre
  measures "d111" distance from line of L1 A0.centre
extrude "Выдавливание26" cut sketch "Эскиз43" against normal blind 10
sketch "Эскиз44" plane through (500, 0, 130) normal (1, 0, 0) x (0, 0, -1)
  circle A0 centre (180, 50) radius 14.5
  line L0 (0, 0) -> (280, 0) projected
  line L1 (280, 0) -> (280, 760) projected
  point P0 (130, 0)
  dimension "d114" = 29
  dimension "d115" = 50
  dimension "d116" = 100
  constraints: 1 centre point
  measures "d114" diameter of A0
  measures "d115" distance from line of L0 A0.centre
  measures "d116" distance from line of L1 A0.centre
extrude "Выдавливание27" cut sketch "Эскиз44" against normal blind 10
sketch "Эскиз45" plane through (500, 0, 130) normal (1, 0, 0) x (0, 0, -1)
  circle A0 centre (130, 700) radius 11.5
  line L0 (280, 0) -> (280, 760) projected
  line L1 (0, 760) -> (280, 760) projected
  point P0 (130, 0)
  dimension "d119" = 23
  dimension "d120" = 150
  dimension "d121" = 60
  constraints: 1 centre point
  measures "d119" diameter of A0
  measures "d120" distance from line of L0 A0.centre
  measures "d121" distance from line of L1 A0.centre
extrude "Выдавливание28" cut sketch "Эскиз45" against normal blind 10
sketch "Эскиз46" plane through (500, 0, 130) normal (1, 0, 0) x (0, 0, -1)
  circle A0 centre (60, 50) radius 11.5
  line L0 (280, 0) -> (280, 760) projected
  point P0 (130, 0)
  dimension "d124" = 23
  dimension "d125" = 220
  constraints: 1 centre point
  measures "d124" diameter of A0
  measures "d125" distance from line of L0 A0.centre
extrude "Выдавливание29" cut sketch "Эскиз46" against normal blind 10
body "Solid1"
